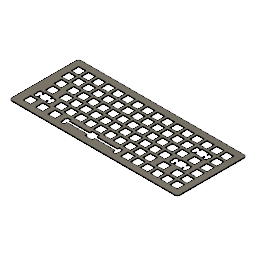
plate (Autodesk Fusion 360 design; units mm, degrees)
Autodesk Fusion 360 part; units mm, degrees
sketch "Sketch1" plane through (0, 0, 0) normal (0, 1, 0) x (1, 0, 0)
  line L0 (1.2912, 1.8259) -> (1.0487, 2.1346)
  line L1 (1.0487, 2.1346) -> (0.831, 2.4612)
  line L2 (0.831, 2.4612) -> (0.6394, 2.8043)
  line L3 (0.6394, 2.8043) -> (0.4754, 3.1598)
  line L4 (0.1557, 4.2912) -> (0.1102, 4.6812)
  line L5 (0.339, 3.5278) -> (0.2329, 3.9067)
  line L6 (0.2329, 3.9067) -> (0.1557, 4.2912)
  line L7 (0.1102, 4.6812) -> (0.0937, 5.0739)
  line L8 (0.4754, 3.1598) -> (0.339, 3.5278)
  line L9 (0.1102, 129.767) -> (0.1557, 130.157)
  line L10 (2.1553, 133.42) -> (2.4819, 133.638)
  line L11 (3.1805, 133.993) -> (3.5485, 134.13)
  line L12 (3.5485, 134.13) -> (3.9274, 134.236)
  line L13 (0.1557, 130.157) -> (0.2329, 130.542)
  line L14 (4.3119, 134.313) -> (4.7019, 134.359)
  line L15 (187.687, 25.1299) -> (187.687, 21.8998)
  line L16 (87.6875, 12.8295) -> (89.4126, 12.8295)
  line L17 (87.6875, 19.0996) -> (87.6875, 12.8295)
  line L18 (0.2329, 130.542) -> (0.339, 130.92)
  line L19 (195.263, 21.8998) -> (194.438, 21.8998)
  line L20 (1.0487, 132.314) -> (1.2912, 132.623)
  line L21 (187.687, 12.8295) -> (189.413, 12.8295)
  line L22 (94.4383, 21.8998) -> (94.4383, 25.1299)
  line L23 (194.438, 12.8295) -> (194.438, 19.0996)
  line L24 (0.339, 130.92) -> (0.4754, 131.288)
  line L25 (0.0951, 129.374) -> (0.1102, 129.767)
  line L26 (0.4754, 131.288) -> (0.6394, 131.644)
  line L27 (134.063, 12.6008) -> (148.063, 12.6008)
  line L28 (15.0013, 12.6008) -> (15.0013, 26.6003)
  line L29 (255.22, 26.6003) -> (255.22, 12.6008)
  line L30 (203.12, 26.6003) -> (217.12, 26.6003)
  line L31 (0.6394, 131.644) -> (0.831, 131.987)
  line L32 (52.8133, 26.6003) -> (52.8133, 12.6008)
  line L33 (2.4819, 133.638) -> (2.825, 133.829)
  line L34 (217.12, 12.6008) -> (203.12, 12.6008)
  line L35 (2.825, 133.829) -> (3.1805, 133.993)
  line L36 (222.17, 12.6008) -> (222.17, 26.6003)
  line L37 (255.22, 12.6008) -> (241.22, 12.6008)
  line L38 (241.22, 12.6008) -> (241.22, 26.6003)
  line L39 (203.12, 12.6008) -> (203.12, 26.6003)
  line L40 (1.2912, 132.623) -> (1.5586, 132.91)
  line L41 (0.831, 131.987) -> (1.0487, 132.314)
  line L42 (222.17, 26.6003) -> (236.17, 26.6003)
  line L43 (134.063, 17.2999) -> (134.063, 12.6008)
  line L44 (1.8466, 133.178) -> (2.1553, 133.42)
  line L45 (3.9274, 134.236) -> (4.3119, 134.313)
  line L46 (187.687, 17.2999) -> (187.687, 12.8295)
  line L47 (0.0937, 5.0739) -> (0.0951, 129.374)
  line L48 (1.5586, 132.91) -> (1.8466, 133.178)
  line L49 (92.7132, 12.8295) -> (94.4383, 12.8295)
  line L50 (94.4383, 25.1299) -> (87.6875, 25.1299)
  line L51 (192.713, 12.8295) -> (194.438, 12.8295)
  line L52 (15.0013, 26.6003) -> (29.0008, 26.6003)
  line L53 (86.8634, 19.0996) -> (87.6875, 19.0996)
  line L54 (87.6875, 25.1299) -> (87.6875, 21.8998)
  line L55 (38.8126, 26.6003) -> (52.8133, 26.6003)
  line L56 (62.6262, 26.6003) -> (76.6258, 26.6003)
  line L57 (94.4383, 12.8295) -> (94.4383, 17.2999)
  line L58 (76.6258, 12.6008) -> (62.6262, 12.6008)
  line L59 (29.0008, 26.6003) -> (29.0008, 12.6008)
  line L60 (87.6875, 21.8998) -> (86.8634, 21.8998)
  line L61 (148.063, 12.6008) -> (148.063, 17.2999)
  line L62 (189.413, 12.8295) -> (189.413, 11.6307)
  line L63 (89.4126, 11.6307) -> (92.7132, 11.6307)
  line L64 (4.7019, 134.359) -> (5.0946, 134.375)
  line L65 (52.8133, 12.6008) -> (38.8126, 12.6008)
  line L66 (89.4126, 12.8295) -> (89.4126, 11.6307)
  line L67 (189.413, 11.6307) -> (192.713, 11.6307)
  line L68 (187.687, 21.8998) -> (148.063, 21.8998)
  line L69 (62.6262, 12.6008) -> (62.6262, 26.6003)
  line L70 (86.8634, 21.8998) -> (86.8634, 19.0996)
  line L71 (134.063, 26.6003) -> (134.063, 21.8998)
  line L72 (15.4258, 38.1497) -> (16.2512, 38.1497)
  line L73 (134.063, 21.8998) -> (94.4383, 21.8998)
  line L74 (194.438, 25.1299) -> (187.687, 25.1299)
  line L75 (74.5314, 45.6487) -> (88.5321, 45.6487)
  line L76 (192.713, 11.6307) -> (192.713, 12.8295)
  line L77 (29.0008, 12.6008) -> (15.0013, 12.6008)
  line L78 (126.632, 31.6494) -> (112.631, 31.6494)
  line L79 (112.631, 31.6494) -> (112.631, 45.6487)
  line L80 (131.681, 45.6487) -> (145.682, 45.6487)
  line L81 (94.4383, 17.2999) -> (134.063, 17.2999)
  line L82 (148.063, 21.8998) -> (148.063, 26.6003)
  line L83 (194.438, 19.0996) -> (195.263, 19.0996)
  line L84 (260.27, 26.6003) -> (274.27, 26.6003)
  line L85 (5.0946, 134.375) -> (319.896, 134.374)
  line L86 (217.12, 26.6003) -> (217.12, 12.6008)
  line L87 (274.27, 26.6003) -> (274.27, 12.6008)
  line L88 (76.6258, 26.6003) -> (76.6258, 12.6008)
  line L89 (92.7132, 11.6307) -> (92.7132, 12.8295)
  line L90 (148.063, 17.2999) -> (187.687, 17.2999)
  line L91 (194.438, 21.8998) -> (194.438, 25.1299)
  line L92 (236.17, 26.6003) -> (236.17, 12.6008)
  line L93 (195.263, 19.0996) -> (195.263, 21.8998)
  line L94 (241.22, 26.6003) -> (255.22, 26.6003)
  line L95 (38.8126, 12.6008) -> (38.8126, 26.6003)
  line L96 (236.17, 12.6008) -> (222.17, 12.6008)
  line L97 (148.063, 26.6003) -> (134.063, 26.6003)
  line L98 (16.2512, 38.1497) -> (16.2512, 31.8795)
  line L99 (40.0512, 44.1798) -> (40.0512, 40.9497)
  line L100 (46.8009, 44.1798) -> (40.0512, 44.1798)
  line L101 (107.582, 31.6494) -> (93.5814, 31.6494)
  line L102 (21.2755, 30.6792) -> (21.2755, 31.8795)
  line L103 (16.2512, 44.1798) -> (16.2512, 40.9497)
  line L104 (17.9751, 31.8795) -> (17.9751, 30.6792)
  line L105 (15.4258, 40.9497) -> (15.4258, 38.1497)
  line L106 (88.5321, 31.6494) -> (74.5314, 31.6494)
  line L107 (93.5814, 45.6487) -> (107.582, 45.6487)
  line L108 (47.6264, 40.9497) -> (46.8009, 40.9497)
  line L109 (38.5258, 31.6494) -> (38.5258, 36.3499)
  line L110 (16.2512, 40.9497) -> (15.4258, 40.9497)
  line L111 (47.6264, 38.1497) -> (47.6264, 40.9497)
  line L112 (23.0008, 40.9497) -> (23.0008, 44.1798)
  line L113 (279.32, 12.6008) -> (279.32, 26.6003)
  line L114 (46.8009, 40.9497) -> (46.8009, 44.1798)
  line L115 (38.5258, 45.6487) -> (24.5263, 45.6487)
  line L116 (24.5263, 45.6487) -> (24.5263, 40.9497)
  line L117 (23.0008, 44.1798) -> (16.2512, 44.1798)
  line L118 (55.4814, 45.6487) -> (69.4821, 45.6487)
  line L119 (69.4821, 45.6487) -> (69.4821, 31.6494)
  line L120 (74.5314, 31.6494) -> (74.5314, 45.6487)
  line L121 (293.32, 26.6003) -> (293.32, 12.6008)
  line L122 (40.0512, 36.3499) -> (40.0512, 31.8795)
  line L123 (24.5263, 40.9497) -> (23.0008, 40.9497)
  line L124 (145.682, 45.6487) -> (145.682, 31.6494)
  line L125 (260.27, 12.6008) -> (260.27, 26.6003)
  line L126 (24.5263, 31.6494) -> (38.5258, 31.6494)
  line L127 (88.5321, 45.6487) -> (88.5321, 31.6494)
  line L128 (45.0755, 31.8795) -> (46.8009, 31.8795)
  line L129 (40.0512, 31.8795) -> (41.7752, 31.8795)
  line L130 (40.0512, 40.9497) -> (38.5258, 40.9497)
  line L131 (38.5258, 36.3499) -> (40.0512, 36.3499)
  line L132 (293.32, 12.6008) -> (279.32, 12.6008)
  line L133 (24.5263, 36.3499) -> (24.5263, 31.6494)
  line L134 (312.37, 12.6008) -> (298.37, 12.6008)
  line L135 (274.27, 12.6008) -> (260.27, 12.6008)
  line L136 (298.37, 26.6003) -> (312.37, 26.6003)
  line L137 (17.9751, 30.6792) -> (21.2755, 30.6792)
  line L138 (46.8009, 38.1497) -> (47.6264, 38.1497)
  line L139 (107.582, 45.6487) -> (107.582, 31.6494)
  line L140 (23.0008, 36.3499) -> (24.5263, 36.3499)
  line L141 (16.2512, 31.8795) -> (17.9751, 31.8795)
  line L142 (23.0008, 31.8795) -> (23.0008, 36.3499)
  line L143 (279.32, 26.6003) -> (293.32, 26.6003)
  line L144 (21.2755, 31.8795) -> (23.0008, 31.8795)
  line L145 (298.37, 12.6008) -> (298.37, 26.6003)
  line L146 (41.7752, 30.6792) -> (45.0755, 30.6792)
  line L147 (69.4821, 31.6494) -> (55.4814, 31.6494)
  line L148 (41.7752, 31.8795) -> (41.7752, 30.6792)
  line L149 (312.37, 26.6003) -> (312.37, 12.6008)
  line L150 (282.937, 50.9295) -> (284.663, 50.9295)
  line L151 (207.881, 31.6494) -> (207.881, 45.6487)
  line L152 (281.413, 55.3999) -> (282.937, 55.3999)
  line L153 (298.37, 31.6494) -> (298.37, 45.6487)
  line L154 (267.126, 45.6487) -> (267.126, 31.6494)
  line L155 (312.37, 31.6494) -> (298.37, 31.6494)
  line L156 (164.732, 45.6487) -> (164.732, 31.6494)
  line L157 (260.863, 50.9295) -> (260.863, 49.7293)
  line L158 (290.513, 57.1997) -> (290.513, 59.9997)
  line L159 (287.963, 49.7293) -> (287.963, 50.9295)
  line L160 (279.32, 45.6487) -> (293.32, 45.6487)
  line L161 (169.781, 31.6494) -> (169.781, 45.6487)
  line L162 (93.5814, 31.6494) -> (93.5814, 45.6487)
  line L163 (55.4814, 31.6494) -> (55.4814, 45.6487)
  line L164 (45.0755, 30.6792) -> (45.0755, 31.8795)
  line L165 (164.732, 31.6494) -> (150.731, 31.6494)
  line L166 (267.126, 31.6494) -> (253.126, 31.6494)
  line L167 (264.163, 50.9295) -> (265.888, 50.9295)
  line L168 (131.681, 31.6494) -> (131.681, 45.6487)
  line L169 (226.931, 45.6487) -> (240.932, 45.6487)
  line L170 (265.888, 55.3999) -> (267.413, 55.3999)
  line L171 (282.937, 55.3999) -> (282.937, 50.9295)
  line L172 (46.8009, 31.8795) -> (46.8009, 38.1497)
  line L173 (221.882, 45.6487) -> (221.882, 31.6494)
  line L174 (188.831, 45.6487) -> (202.832, 45.6487)
  line L175 (253.126, 45.6487) -> (267.126, 45.6487)
  line L176 (293.32, 45.6487) -> (293.32, 31.6494)
  line L177 (265.888, 50.9295) -> (265.888, 55.3999)
  line L178 (260.863, 49.7293) -> (264.163, 49.7293)
  line L179 (267.413, 55.3999) -> (267.413, 50.6995)
  line L180 (281.413, 50.6995) -> (281.413, 55.3999)
  line L181 (293.32, 31.6494) -> (279.32, 31.6494)
  line L182 (150.731, 31.6494) -> (150.731, 45.6487)
  line L183 (183.782, 45.6487) -> (183.782, 31.6494)
  line L184 (258.313, 57.1997) -> (259.137, 57.1997)
  line L185 (169.781, 45.6487) -> (183.782, 45.6487)
  line L186 (289.687, 57.1997) -> (290.513, 57.1997)
  line L187 (126.632, 45.6487) -> (126.632, 31.6494)
  line L188 (290.513, 59.9997) -> (289.687, 59.9997)
  line L189 (289.687, 50.9295) -> (289.687, 57.1997)
  line L190 (287.963, 50.9295) -> (289.687, 50.9295)
  line L191 (258.313, 59.9997) -> (258.313, 57.1997)
  line L192 (202.832, 31.6494) -> (188.831, 31.6494)
  line L193 (112.631, 45.6487) -> (126.632, 45.6487)
  line L194 (38.5258, 40.9497) -> (38.5258, 45.6487)
  line L195 (284.663, 49.7293) -> (287.963, 49.7293)
  line L196 (240.932, 45.6487) -> (240.932, 31.6494)
  line L197 (226.931, 31.6494) -> (226.931, 45.6487)
  line L198 (202.832, 45.6487) -> (202.832, 31.6494)
  line L199 (98.0571, 64.6987) -> (98.0571, 50.6995)
  line L200 (212.357, 50.6995) -> (198.356, 50.6995)
  line L201 (264.163, 49.7293) -> (264.163, 50.9295)
  line L202 (240.932, 31.6494) -> (226.931, 31.6494)
  line L203 (281.413, 64.6987) -> (267.413, 64.6987)
  line L204 (183.782, 31.6494) -> (169.781, 31.6494)
  line L205 (193.307, 50.6995) -> (179.306, 50.6995)
  line L206 (98.0571, 50.6995) -> (84.0564, 50.6995)
  line L207 (259.137, 50.9295) -> (260.863, 50.9295)
  line L208 (33.7633, 64.6987) -> (33.7633, 50.6995)
  line L209 (312.37, 64.6987) -> (312.37, 50.6995)
  line L210 (31.3821, 69.7495) -> (17.3812, 69.7495)
  line L211 (312.37, 50.6995) -> (298.37, 50.6995)
  line L212 (217.406, 64.6987) -> (231.407, 64.6987)
  line L213 (79.0071, 50.6995) -> (65.0064, 50.6995)
  line L214 (217.406, 50.6995) -> (217.406, 64.6987)
  line L215 (265.888, 63.2298) -> (259.137, 63.2298)
  line L216 (265.888, 59.9997) -> (265.888, 63.2298)
  line L217 (79.0071, 64.6987) -> (79.0071, 50.6995)
  line L218 (160.256, 64.6987) -> (174.257, 64.6987)
  line L219 (259.137, 57.1997) -> (259.137, 50.9295)
  line L220 (145.682, 31.6494) -> (131.681, 31.6494)
  line L221 (298.37, 45.6487) -> (312.37, 45.6487)
  line L222 (221.882, 31.6494) -> (207.881, 31.6494)
  line L223 (150.731, 45.6487) -> (164.732, 45.6487)
  line L224 (188.831, 31.6494) -> (188.831, 45.6487)
  line L225 (231.407, 64.6987) -> (231.407, 50.6995)
  line L226 (253.126, 31.6494) -> (253.126, 45.6487)
  line L227 (259.137, 63.2298) -> (259.137, 59.9997)
  line L228 (284.663, 50.9295) -> (284.663, 49.7293)
  line L229 (259.137, 59.9997) -> (258.313, 59.9997)
  line L230 (267.413, 50.6995) -> (281.413, 50.6995)
  line L231 (231.407, 50.6995) -> (217.406, 50.6995)
  line L232 (298.37, 64.6987) -> (312.37, 64.6987)
  line L233 (198.356, 50.6995) -> (198.356, 64.6987)
  line L234 (136.157, 50.6995) -> (122.156, 50.6995)
  line L235 (267.413, 64.6987) -> (267.413, 59.9997)
  line L236 (59.9556, 64.6987) -> (59.9556, 50.6995)
  line L237 (279.32, 31.6494) -> (279.32, 45.6487)
  line L238 (155.207, 50.6995) -> (141.206, 50.6995)
  line L239 (33.7633, 50.6995) -> (19.7624, 50.6995)
  line L240 (250.457, 64.6987) -> (250.457, 50.6995)
  line L241 (267.413, 59.9997) -> (265.888, 59.9997)
  line L242 (312.37, 45.6487) -> (312.37, 31.6494)
  line L243 (236.456, 64.6987) -> (250.457, 64.6987)
  line L244 (250.457, 50.6995) -> (236.456, 50.6995)
  line L245 (19.7624, 50.6995) -> (19.7624, 64.6987)
  line L246 (122.156, 64.6987) -> (136.157, 64.6987)
  line L247 (207.881, 45.6487) -> (221.882, 45.6487)
  line L248 (117.107, 50.6995) -> (103.106, 50.6995)
  line L249 (298.37, 50.6995) -> (298.37, 64.6987)
  line L250 (155.207, 64.6987) -> (155.207, 50.6995)
  line L251 (174.545, 69.7495) -> (174.545, 83.7487)
  line L252 (269.795, 102.799) -> (269.795, 98.0997)
  line L253 (207.595, 83.7487) -> (207.595, 69.7495)
  line L254 (103.106, 64.6987) -> (117.107, 64.6987)
  line L255 (198.356, 64.6987) -> (212.357, 64.6987)
  line L256 (298.37, 83.7487) -> (312.37, 83.7487)
  line L257 (79.2949, 83.7487) -> (93.2946, 83.7487)
  line L258 (17.3812, 83.7487) -> (31.3821, 83.7487)
  line L259 (122.156, 50.6995) -> (122.156, 64.6987)
  line L260 (212.645, 83.7487) -> (226.645, 83.7487)
  line L261 (55.1946, 83.7487) -> (55.1946, 69.7495)
  line L262 (84.0564, 50.6995) -> (84.0564, 64.6987)
  line L263 (207.595, 69.7495) -> (193.595, 69.7495)
  line L264 (55.1946, 69.7495) -> (41.1949, 69.7495)
  line L265 (65.0064, 64.6987) -> (79.0071, 64.6987)
  line L266 (179.306, 64.6987) -> (193.307, 64.6987)
  line L267 (212.357, 64.6987) -> (212.357, 50.6995)
  line L268 (289.687, 63.2298) -> (282.937, 63.2298)
  line L269 (169.495, 69.7495) -> (155.495, 69.7495)
  line L270 (231.695, 69.7495) -> (231.695, 83.7487)
  line L271 (45.9564, 50.6995) -> (45.9564, 64.6987)
  line L272 (268.27, 98.0997) -> (268.27, 101.33)
  line L273 (261.52, 101.33) -> (261.52, 98.0997)
  line L274 (65.0064, 50.6995) -> (65.0064, 64.6987)
  line L275 (236.456, 50.6995) -> (236.456, 64.6987)
  line L276 (41.1949, 83.7487) -> (55.1946, 83.7487)
  line L277 (19.7624, 64.6987) -> (33.7633, 64.6987)
  line L278 (136.157, 64.6987) -> (136.157, 50.6995)
  line L279 (174.257, 50.6995) -> (160.256, 50.6995)
  line L280 (289.687, 59.9997) -> (289.687, 63.2298)
  line L281 (282.937, 63.2298) -> (282.937, 59.9997)
  line L282 (226.645, 69.7495) -> (212.645, 69.7495)
  line L283 (112.345, 83.7487) -> (112.345, 69.7495)
  line L284 (150.445, 69.7495) -> (136.445, 69.7495)
  line L285 (174.257, 64.6987) -> (174.257, 50.6995)
  line L286 (193.307, 64.6987) -> (193.307, 50.6995)
  line L287 (281.413, 59.9997) -> (281.413, 64.6987)
  line L288 (59.9556, 50.6995) -> (45.9564, 50.6995)
  line L289 (141.206, 50.6995) -> (141.206, 64.6987)
  line L290 (179.306, 50.6995) -> (179.306, 64.6987)
  line L291 (117.107, 64.6987) -> (117.107, 50.6995)
  line L292 (84.0564, 64.6987) -> (98.0571, 64.6987)
  line L293 (31.3821, 83.7487) -> (31.3821, 69.7495)
  line L294 (45.9564, 64.6987) -> (59.9556, 64.6987)
  line L295 (282.937, 59.9997) -> (281.413, 59.9997)
  line L296 (17.3812, 69.7495) -> (17.3812, 83.7487)
  line L297 (103.106, 50.6995) -> (103.106, 64.6987)
  line L298 (141.206, 64.6987) -> (155.207, 64.6987)
  line L299 (160.256, 50.6995) -> (160.256, 64.6987)
  line L300 (136.445, 69.7495) -> (136.445, 83.7487)
  line L301 (74.2446, 69.7495) -> (60.2449, 69.7495)
  line L302 (74.2446, 83.7487) -> (74.2446, 69.7495)
  line L303 (245.695, 83.7487) -> (245.695, 69.7495)
  line L304 (261.52, 95.2997) -> (261.52, 89.0295)
  line L305 (131.395, 69.7495) -> (117.395, 69.7495)
  line L306 (288.557, 69.7495) -> (274.556, 69.7495)
  line L307 (288.557, 83.7487) -> (288.557, 69.7495)
  line L308 (136.445, 83.7487) -> (150.445, 83.7487)
  line L309 (250.745, 69.7495) -> (250.745, 83.7487)
  line L310 (269.795, 98.0997) -> (268.27, 98.0997)
  line L311 (117.395, 69.7495) -> (117.395, 83.7487)
  line L312 (231.695, 83.7487) -> (245.695, 83.7487)
  line L313 (155.495, 83.7487) -> (169.495, 83.7487)
  line L314 (212.645, 69.7495) -> (212.645, 83.7487)
  line L315 (261.52, 98.0997) -> (260.695, 98.0997)
  line L316 (98.3449, 83.7487) -> (112.345, 83.7487)
  line L317 (261.52, 89.0295) -> (263.245, 89.0295)
  line L318 (312.37, 83.7487) -> (312.37, 69.7495)
  line L319 (245.695, 69.7495) -> (231.695, 69.7495)
  line L320 (98.3449, 69.7495) -> (98.3449, 83.7487)
  line L321 (250.745, 83.7487) -> (264.745, 83.7487)
  line L322 (260.695, 95.2997) -> (261.52, 95.2997)
  line L323 (264.745, 83.7487) -> (264.745, 69.7495)
  line L324 (60.2449, 83.7487) -> (74.2446, 83.7487)
  line L325 (312.37, 69.7495) -> (298.37, 69.7495)
  line L326 (274.556, 69.7495) -> (274.556, 83.7487)
  line L327 (41.1949, 69.7495) -> (41.1949, 83.7487)
  line L328 (298.37, 69.7495) -> (298.37, 83.7487)
  line L329 (193.595, 83.7487) -> (207.595, 83.7487)
  line L330 (60.2449, 69.7495) -> (60.2449, 83.7487)
  line L331 (188.545, 69.7495) -> (174.545, 69.7495)
  line L332 (264.745, 69.7495) -> (250.745, 69.7495)
  line L333 (79.2949, 69.7495) -> (79.2949, 83.7487)
  line L334 (169.495, 83.7487) -> (169.495, 69.7495)
  line L335 (131.395, 83.7487) -> (131.395, 69.7495)
  line L336 (117.395, 83.7487) -> (131.395, 83.7487)
  line L337 (226.645, 83.7487) -> (226.645, 69.7495)
  line L338 (112.345, 69.7495) -> (98.3449, 69.7495)
  line L339 (150.445, 83.7487) -> (150.445, 69.7495)
  line L340 (93.2946, 83.7487) -> (93.2946, 69.7495)
  line L341 (174.545, 83.7487) -> (188.545, 83.7487)
  line L342 (260.695, 98.0997) -> (260.695, 95.2997)
  line L343 (193.595, 69.7495) -> (193.595, 83.7487)
  line L344 (93.2946, 69.7495) -> (79.2949, 69.7495)
  line L345 (155.495, 69.7495) -> (155.495, 83.7487)
  line L346 (268.27, 101.33) -> (261.52, 101.33)
  line L347 (274.556, 83.7487) -> (288.557, 83.7487)
  line L348 (102.82, 102.799) -> (102.82, 88.7995)
  line L349 (50.7199, 102.799) -> (64.7196, 102.799)
  line L350 (285.32, 93.4999) -> (285.32, 89.0295)
  line L351 (198.07, 102.799) -> (198.07, 88.7995)
  line L352 (283.795, 98.0997) -> (283.795, 102.799)
  line L353 (140.92, 88.7995) -> (126.92, 88.7995)
  line L354 (283.795, 102.799) -> (269.795, 102.799)
  line L355 (50.7199, 88.7995) -> (50.7199, 102.799)
  line L356 (121.868, 102.799) -> (121.868, 88.7995)
  line L357 (263.245, 89.0295) -> (263.245, 87.8293)
  line L358 (45.6696, 88.7995) -> (31.6701, 88.7995)
  line L359 (268.27, 93.4999) -> (269.795, 93.4999)
  line L360 (283.795, 88.7995) -> (283.795, 93.4999)
  line L361 (64.7196, 88.7995) -> (50.7199, 88.7995)
  line L362 (88.8199, 88.7995) -> (88.8199, 102.799)
  line L363 (145.97, 88.7995) -> (145.97, 102.799)
  line L364 (165.02, 88.7995) -> (165.02, 102.799)
  line L365 (179.02, 102.799) -> (179.02, 88.7995)
  line L366 (102.82, 88.7995) -> (88.8199, 88.7995)
  line L367 (126.92, 88.7995) -> (126.92, 102.799)
  line L368 (145.97, 102.799) -> (159.97, 102.799)
  line L369 (285.32, 98.0997) -> (283.795, 98.0997)
  line L370 (69.7699, 102.799) -> (83.7696, 102.799)
  line L371 (159.97, 88.7995) -> (145.97, 88.7995)
  line L372 (179.02, 88.7995) -> (165.02, 88.7995)
  line L373 (64.7196, 102.799) -> (64.7196, 88.7995)
  line L374 (269.795, 88.7995) -> (283.795, 88.7995)
  line L375 (45.6696, 102.799) -> (45.6696, 88.7995)
  line L376 (107.869, 88.7995) -> (107.869, 102.799)
  line L377 (292.895, 98.0997) -> (292.07, 98.0997)
  line L378 (266.544, 87.8293) -> (266.544, 89.0295)
  line L379 (31.6701, 102.799) -> (45.6696, 102.799)
  line L380 (269.795, 93.4999) -> (269.795, 88.7995)
  line L381 (26.6196, 88.7995) -> (12.6201, 88.7995)
  line L382 (283.795, 93.4999) -> (285.32, 93.4999)
  line L383 (287.045, 89.0295) -> (287.045, 87.8293)
  line L384 (121.868, 88.7995) -> (107.869, 88.7995)
  line L385 (290.344, 89.0295) -> (292.07, 89.0295)
  line L386 (188.545, 83.7487) -> (188.545, 69.7495)
  line L387 (31.6701, 88.7995) -> (31.6701, 102.799)
  line L388 (285.32, 101.33) -> (285.32, 98.0997)
  line L389 (69.7699, 88.7995) -> (69.7699, 102.799)
  line L390 (266.544, 89.0295) -> (268.27, 89.0295)
  line L391 (287.045, 87.8293) -> (290.344, 87.8293)
  line L392 (83.7696, 88.7995) -> (69.7699, 88.7995)
  line L393 (126.92, 102.799) -> (140.92, 102.799)
  line L394 (165.02, 102.799) -> (179.02, 102.799)
  line L395 (12.6201, 102.799) -> (26.6196, 102.799)
  line L396 (292.07, 89.0295) -> (292.07, 95.2997)
  line L397 (159.97, 102.799) -> (159.97, 88.7995)
  line L398 (203.12, 107.849) -> (203.12, 121.849)
  line L399 (126.92, 107.849) -> (126.92, 121.849)
  line L400 (12.6201, 121.849) -> (26.6196, 121.849)
  line L401 (241.22, 88.7995) -> (241.22, 102.799)
  line L402 (26.6196, 102.799) -> (26.6196, 88.7995)
  line L403 (12.6201, 88.7995) -> (12.6201, 102.799)
  line L404 (107.869, 107.849) -> (107.869, 121.849)
  line L405 (222.17, 88.7995) -> (222.17, 102.799)
  line L406 (69.7699, 107.849) -> (69.7699, 121.849)
  line L407 (222.17, 121.849) -> (236.17, 121.849)
  line L408 (165.02, 121.849) -> (179.02, 121.849)
  line L409 (12.6201, 107.849) -> (12.6201, 121.849)
  line L410 (107.869, 102.799) -> (121.868, 102.799)
  line L411 (312.37, 88.7995) -> (298.37, 88.7995)
  line L412 (203.12, 102.799) -> (217.12, 102.799)
  line L413 (121.868, 121.849) -> (121.868, 107.849)
  line L414 (298.37, 88.7995) -> (298.37, 102.799)
  line L415 (198.07, 121.849) -> (198.07, 107.849)
  line L416 (292.07, 95.2997) -> (292.895, 95.2997)
  line L417 (83.7696, 102.799) -> (83.7696, 88.7995)
  line L418 (268.27, 89.0295) -> (268.27, 93.4999)
  line L419 (236.17, 121.849) -> (236.17, 107.849)
  line L420 (285.32, 89.0295) -> (287.045, 89.0295)
  line L421 (140.92, 102.799) -> (140.92, 88.7995)
  line L422 (292.895, 95.2997) -> (292.895, 98.0997)
  line L423 (217.12, 107.849) -> (203.12, 107.849)
  line L424 (184.07, 88.7995) -> (184.07, 102.799)
  line L425 (298.37, 102.799) -> (312.37, 102.799)
  line L426 (145.97, 121.849) -> (159.97, 121.849)
  line L427 (64.7196, 107.849) -> (50.7199, 107.849)
  line L428 (263.245, 87.8293) -> (266.544, 87.8293)
  line L429 (217.12, 88.7995) -> (203.12, 88.7995)
  line L430 (292.07, 98.0997) -> (292.07, 101.33)
  line L431 (179.02, 107.849) -> (165.02, 107.849)
  line L432 (290.344, 87.8293) -> (290.344, 89.0295)
  line L433 (88.8199, 121.849) -> (102.82, 121.849)
  line L434 (145.97, 107.849) -> (145.97, 121.849)
  line L435 (203.12, 121.849) -> (217.12, 121.849)
  line L436 (107.869, 121.849) -> (121.868, 121.849)
  line L437 (159.97, 107.849) -> (145.97, 107.849)
  line L438 (88.8199, 102.799) -> (102.82, 102.799)
  line L439 (159.97, 121.849) -> (159.97, 107.849)
  line L440 (83.7696, 107.849) -> (69.7699, 107.849)
  line L441 (292.07, 101.33) -> (285.32, 101.33)
  line L442 (102.82, 121.849) -> (102.82, 107.849)
  line L443 (184.07, 107.849) -> (184.07, 121.849)
  line L444 (236.17, 102.799) -> (236.17, 88.7995)
  line L445 (165.02, 107.849) -> (165.02, 121.849)
  line L446 (179.02, 121.849) -> (179.02, 107.849)
  line L447 (184.07, 102.799) -> (198.07, 102.799)
  line L448 (140.92, 107.849) -> (126.92, 107.849)
  line L449 (241.22, 102.799) -> (255.22, 102.799)
  line L450 (83.7696, 121.849) -> (83.7696, 107.849)
  line L451 (324.159, 2.4612) -> (323.941, 2.1346)
  line L452 (50.7199, 121.849) -> (64.7196, 121.849)
  line L453 (324.757, 130.542) -> (324.834, 130.157)
  line L454 (324.834, 130.157) -> (324.879, 129.767)
  line L455 (324.879, 4.6812) -> (324.834, 4.2912)
  line L456 (312.37, 102.799) -> (312.37, 88.7995)
  line L457 (323.698, 1.8259) -> (323.431, 1.5379)
  line L458 (255.22, 88.7995) -> (241.22, 88.7995)
  line L459 (45.6696, 107.849) -> (31.6701, 107.849)
  line L460 (324.35, 2.8043) -> (324.159, 2.4612)
  line L461 (323.941, 2.1346) -> (323.698, 1.8259)
  line L462 (322.834, 1.028) -> (322.508, 0.8103)
  line L463 (321.809, 133.993) -> (322.165, 133.829)
  line L464 (31.6701, 121.849) -> (45.6696, 121.849)
  line L465 (222.17, 102.799) -> (236.17, 102.799)
  line L466 (140.92, 121.849) -> (140.92, 107.849)
  line L467 (126.92, 121.849) -> (140.92, 121.849)
  line L468 (198.07, 107.849) -> (184.07, 107.849)
  line L469 (217.12, 102.799) -> (217.12, 88.7995)
  line L470 (31.6701, 107.849) -> (31.6701, 121.849)
  line L471 (64.7196, 121.849) -> (64.7196, 107.849)
  line L472 (236.17, 88.7995) -> (222.17, 88.7995)
  line L473 (102.82, 107.849) -> (88.8199, 107.849)
  line L474 (88.8199, 107.849) -> (88.8199, 121.849)
  line L475 (45.6696, 121.849) -> (45.6696, 107.849)
  line L476 (321.062, 134.236) -> (321.441, 134.13)
  line L477 (198.07, 88.7995) -> (184.07, 88.7995)
  line L478 (323.698, 132.623) -> (323.941, 132.314)
  line L479 (324.879, 129.767) -> (324.895, 129.374)
  line L480 (324.651, 130.92) -> (324.757, 130.542)
  line L481 (50.7199, 107.849) -> (50.7199, 121.849)
  line L482 (26.6196, 121.849) -> (26.6196, 107.849)
  line L483 (121.868, 107.849) -> (107.869, 107.849)
  line L484 (203.12, 88.7995) -> (203.12, 102.799)
  line L485 (26.6196, 107.849) -> (12.6201, 107.849)
  line L486 (69.7699, 121.849) -> (83.7696, 121.849)
  line L487 (217.12, 121.849) -> (217.12, 107.849)
  line L488 (184.07, 121.849) -> (198.07, 121.849)
  line L489 (255.22, 102.799) -> (255.22, 88.7995)
  line L490 (324.896, 5.0726) -> (324.879, 4.6812)
  line L491 (324.834, 4.2912) -> (324.757, 3.9067)
  line L492 (324.651, 3.5278) -> (324.514, 3.1598)
  line L493 (324.514, 3.1598) -> (324.35, 2.8043)
  line L494 (323.431, 1.5379) -> (323.143, 1.2705)
  line L495 (324.895, 129.374) -> (324.896, 5.0726)
  line L496 (324.514, 131.288) -> (324.651, 130.92)
  line L497 (320.678, 0.135) -> (320.288, 0.0896)
  line L498 (322.834, 133.42) -> (323.143, 133.178)
  line L499 (322.508, 133.638) -> (322.834, 133.42)
  line L500 (312.37, 121.849) -> (312.37, 107.849)
  line L501 (255.22, 121.849) -> (255.22, 107.849)
  line L502 (293.32, 121.849) -> (293.32, 107.849)
  line L503 (322.165, 133.829) -> (322.508, 133.638)
  line L504 (324.757, 3.9067) -> (324.651, 3.5278)
  line L505 (321.441, 134.13) -> (321.809, 133.993)
  line L506 (323.941, 132.314) -> (324.159, 131.987)
  line L507 (320.288, 134.359) -> (320.678, 134.313)
  line L508 (323.431, 132.91) -> (323.698, 132.623)
  line L509 (321.441, 0.3183) -> (321.062, 0.2122)
  line L510 (319.896, 0.073) -> (5.0946, 0.073)
  line L511 (320.678, 134.313) -> (321.062, 134.236)
  line L512 (324.35, 131.644) -> (324.514, 131.288)
  line L513 (293.32, 107.849) -> (279.32, 107.849)
  line L514 (274.27, 107.849) -> (260.27, 107.849)
  line L515 (320.288, 0.0896) -> (319.896, 0.073)
  line L516 (324.159, 131.987) -> (324.35, 131.644)
  line L517 (5.0946, 0.073) -> (4.7019, 0.0896)
  line L518 (274.27, 121.849) -> (274.27, 107.849)
  line L519 (319.896, 134.374) -> (320.288, 134.359)
  line L520 (323.143, 1.2706) -> (322.834, 1.028)
  line L521 (322.165, 0.6187) -> (321.809, 0.4548)
  line L522 (260.27, 107.849) -> (260.27, 121.849)
  line L523 (312.37, 107.849) -> (298.37, 107.849)
  line L524 (321.062, 0.2122) -> (320.678, 0.135)
  line L525 (321.809, 0.4548) -> (321.441, 0.3183)
  line L526 (279.32, 107.849) -> (279.32, 121.849)
  line L527 (323.143, 133.178) -> (323.431, 132.91)
  line L528 (298.37, 121.849) -> (312.37, 121.849)
  line L529 (255.22, 107.849) -> (241.22, 107.849)
  line L530 (298.37, 107.849) -> (298.37, 121.849)
  line L531 (260.27, 121.849) -> (274.27, 121.849)
  line L532 (322.508, 0.8103) -> (322.165, 0.6187)
  line L533 (279.32, 121.849) -> (293.32, 121.849)
  line L534 (236.17, 107.849) -> (222.17, 107.849)
  line L535 (222.17, 107.849) -> (222.17, 121.849)
  line L536 (241.22, 121.849) -> (255.22, 121.849)
  line L537 (3.9274, 0.2122) -> (3.5485, 0.3183)
  line L538 (4.7019, 0.0896) -> (4.3119, 0.135)
  line L539 (3.1805, 0.4548) -> (2.825, 0.6187)
  line L540 (2.825, 0.6187) -> (2.4819, 0.8103)
  line L541 (2.4819, 0.8103) -> (2.1553, 1.028)
  line L542 (2.1553, 1.028) -> (1.8466, 1.2706)
  line L543 (1.8466, 1.2706) -> (1.5586, 1.5379)
  line L544 (1.5586, 1.5379) -> (1.2912, 1.8259)
  line L545 (241.22, 107.849) -> (241.22, 121.849)
  line L546 (4.3119, 0.135) -> (3.9274, 0.2122)
  line L547 (3.5485, 0.3183) -> (3.1805, 0.4548)
extrude "Extrude1" add sketch "Sketch1" along normal blind 1.5
